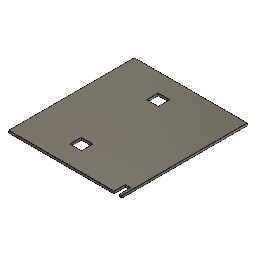
back _buttonv1 (Autodesk Fusion 360 design; units mm, degrees)
Autodesk Fusion 360 part; units mm, degrees
box "BoxPrimitive5" add length 100 width 90 height 2 placed x (0, 0, -1) y (-1, 0, 0) z (0, 1, 0) at (0, 0, 0)
box "BoxPrimitive6" cut length 9 width 4 height -14 placed x (0, 0, 1) y (1, 0, 0) z (0, 1, 0) at (-6, 2, -9)
box "BoxPrimitive7" cut length 9 width 9 height -11 placed x (0, 0, -1) y (-1, 0, 0) z (0, 1, 0) at (-47, 2, -15)
box "BoxPrimitive8" cut length 9 width 9 height -10 placed x (0, 0, -1) y (-1, 0, 0) z (0, 1, 0) at (-47, 2, -76)
